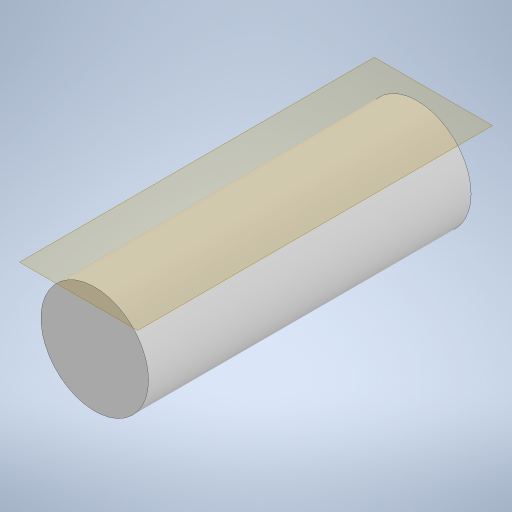
# Autodesk Inventor part: eje_Agujero
Saved by Autodesk Inventor 2023.2 (Build 272271030, 271C)
## iProperties
Created: 2023-10-02
Part Number: eje_Agujero
Material: Generic
Document SubType Name: Modeling
Designer: Cris Pat
Density: 1 g/cm^3
Appearance: Default
Author: Cris Pat
Autodesk Inventor part; units mm, degrees
ref_plane "YZ Plane" through (0, 0, 0) normal (1, 0, 0) x (0, 1, 0)
ref_plane "XY Plane" through (0, 0, 0) normal (0, 0, 1) x (1, 0, 0)
sketch "Sketch1" plane through (0, 0, 0) normal (0, 0, 1) x (1, 0, 0)
  circle A0 centre (0, 0) radius 100.0755
  dimension "d0" = 200
  constraints: 1 centre point, 1 coincident
extrude "Extrusion1" add sketch "Sketch1" along normal blind 600
ref_plane "Work Plane1" through (0, 100.0755, 0) normal (0, 1, 0) x (-1, 0, 0)
equation "\"d0\" = D_agujero"
equation "\"d1\" = 12 * espesor"
equation "\"d3\" = 0"
equation "\"d6\" = 0"
equation "\"D_agujero\" = 200"
equation "\"espesor\" = 50"
body "Solid1"
